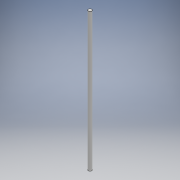
# Autodesk Inventor part: TABLE ROD
Saved by Autodesk Inventor 2018 (Build 220112000, 112)
## iProperties
Created: 2018-10-13
Part Number: TABLE ROD
Material: Generic
Document SubType Name: Modeling
Designer: Matthew Morey
Density: 1 g/cm^3
Appearance: Default
Author: Matthew Morey
Autodesk Inventor part; units mm, degrees
ref_plane "YZ Plane" through (0, 0, 0) normal (1, 0, 0) x (0, 1, 0)
ref_plane "XZ Plane" through (0, 0, 0) normal (0, 1, 0) x (-1, 0, 0)
ref_plane "XY Plane" through (0, 0, 0) normal (0, 0, 1) x (1, 0, 0)
sketch "Sketch1" plane through (0, 0, 0) normal (0, 0, 1) x (1, 0, 0)
  circle A0 centre (0, 0) radius 4
  dimension "d0" = 8
  constraints: 1 centre point, 1 coincident
  measures "d0" diameter of A0
extrude "Extrusion1" add sketch "Sketch1" along normal blind 309.9
chamfer "Chamfer1" distance 0.4 angle 45 2 edges at (-4, 0, 309.9) (-4, 0, 0)
body "Solid1"
